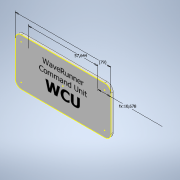
# Autodesk Inventor part: FrontLogo
Saved by Autodesk Inventor 2022 (Build 260153000, 153)
## iProperties
Created: 2021-04-23
Part Number: FrontLogo
Material: Generic
Document SubType Name: Modeling
Designer: Viktor
Density: 1 g/cm^3
Appearance: Default
Author: Viktor
Autodesk Inventor part; units mm, degrees
ref_plane "YZ Plane" through (0, 0, 0) normal (1, 0, 0) x (0, 1, 0)
ref_plane "XZ Plane" through (0, 0, 0) normal (0, 1, 0) x (-1, 0, 0)
ref_plane "XY Plane" through (0, 0, 0) normal (0, 0, 1) x (1, 0, 0)
sketch "Sketch1" plane through (0, 0, 0) normal (0, 0, 1) x (1, 0, 0)
  line L0 (-39.5, -19.5) -> (39.5, -19.5)
  line L1 (39.5, -19.5) -> (39.5, 19.5)
  line L2 (39.5, 19.5) -> (-39.5, 19.5)
  line L3 (-39.5, 19.5) -> (-39.5, -19.5)
  line L4 (-39.5, -19.5) -> (39.5, 19.5) construction
  line L5 (39.5, -19.5) -> (-39.5, 19.5) construction
  point P0 (0, 0)
  dimension "d0" = 79
  dimension "d1" = 39
  constraints: 12 end point, 2 midpoint, 2 parallel, 1 horizontal, 1 perpendicular
  measures "d0" distance of L1.end L2.end
  measures "d1" distance of L0.end L1.end
extrude "Extrusion1" add sketch "Sketch1" along normal blind 2
fillet "Fillet1" radius 5 4 edges at (39.5, -19.5, 1) (39.5, 19.5, 1) (-39.5, 19.5, 1) (-39.5, -19.5, 1)
sketch "Sketch2" plane through (0, 0, 2) normal (0, 0, 1) x (1, 0, 0)
  arc A0 (-39.5, -14.5) -> (-34.5, -19.5) centre (-34.5, -14.5) ccw projected
  line L0 (-34.5, -19.5) -> (34.5, -19.5) projected
  arc A1 (34.5, -19.5) -> (39.5, -14.5) centre (34.5, -14.5) ccw projected
  line L1 (39.5, -14.5) -> (39.5, 14.5) projected
  arc A2 (39.5, 14.5) -> (34.5, 19.5) centre (34.5, 14.5) ccw projected
  line L2 (34.5, 19.5) -> (-34.5, 19.5) projected
  arc A3 (-34.5, 19.5) -> (-39.5, 14.5) centre (-34.5, 14.5) ccw projected
  line L3 (-39.5, 14.5) -> (-39.5, -14.5) projected
  line L4 (-28.8222, 12.3619) -> (28.8222, 12.3619) construction
  line L5 (28.8222, 12.3619) -> (28.8222, -11.0912) construction
  line L6 (28.8222, -11.0912) -> (-28.8222, -11.0912) construction
  line L7 (-28.8222, -11.0912) -> (-28.8222, 12.3619) construction
  point P0 (0, 0)
  dimension "d5" = 57.6443
  dimension "d6" = 79
  dimension "d7" = 10.6778
  constraints: 2 other
  measures "d5" distance between parallel lines of L5 L7
  measures "d6" distance between parallel lines of L1 L3
  measures "d7" distance between parallel lines of L1 L5
equation "\"d7\" = -0.5 * d5 + 0.5 * d6"
body "Solid1"
